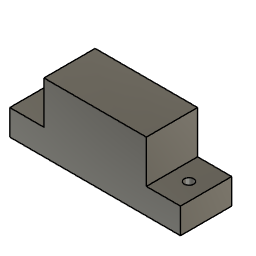
crank-holder (Autodesk Fusion 360 design; units mm, degrees)
Autodesk Fusion 360 part; units mm, degrees
sketch "main" plane through (0, 0, 0) normal (0, 1, 0) x (1, 0, 0) in component "crank-holder"
  line L0 (30, -20) -> (-30, -20)
  line L1 (-30, -20) -> (-30, 20)
  line L2 (-30, 20) -> (30, 20)
  line L3 (30, 20) -> (30, -20)
  line L4 (30, -20) -> (-30, 20) construction
  line L5 (-30, -20) -> (30, 20) construction
  circle A0 centre (0, 0) radius 4.425
  line L6 (-30, 20) -> (-50, 20) construction
  line L7 (-50, 20) -> (50, 20)
  line L8 (50, 20) -> (50, 5)
  line L9 (50, 5) -> (-50, 5)
  line L10 (-50, 5) -> (-50, 20)
  dimension "d1" = 60
  dimension "d2" = 40
  dimension "d3" = 8.85
  dimension "d4" = 20
  dimension "d5" = 100
  dimension "d6" = 15
  constraint horizontal L0
  constraint perpendicular L0 L1
  constraint parallel L0 L2
  constraint parallel L1 L3
  constraint coincident L4 A0.centre
  constraint coincident L5 A0.centre
  constraint coincident A0.centre origin
  constraint perpendicular L1 L6
  constraint horizontal L7
  constraint vertical L8
  constraint horizontal L9
  constraint vertical L10
  measures "d1" distance of L1.end L2.end
  measures "d2" distance of L0.end L1.end
  measures "d3" diameter of A0
  measures "d4" distance of L1.end L6.end
  measures "d5" distance of L6.end L7.end
  measures "d6" distance of L6.end L9.end
extrude "Extrude1" add sketch "main" against normal blind 30 contours L0 L1 L3 L9 | L1 L2 L3 L7 L9 | L3 L7 L8 L9 | L1 L7 L9 L10 | A0 in component "crank-holder"
extrude "Extrude2" add sketch "main" along normal blind 8.5 contours A0 in component "crank-holder"
sketch "screws" plane through (0, 0, -5) normal (0, 0, 1) x (-1, 0, 0) in component "crank-holder"
  line L0 (30, 0) -> (50, 0)
  line L1 (50, 0) -> (50, 30)
  line L2 (50, 30) -> (30, 30)
  line L3 (30, 30) -> (30, 0)
  line L4 (50, 0) -> (30, 30) construction
  line L5 (50, 30) -> (30, 0) construction
  line L6 (-50, 0) -> (-30, 30) construction
  line L7 (-50, 30) -> (-30, 0) construction
  circle A0 centre (40, 15) radius 2.75
  circle A1 centre (-40, 15) radius 2.75
  point P0 (-50, 0)
  point P1 (-30, 30)
  point P2 (-50, 30)
  point P3 (-30, 0)
  dimension "d11" = 5.5
  dimension "d12" = 5.5
  constraint coincident L0.end L1.start
  constraint coincident L2.end L3.start
  constraint coincident L1.end L2.start
  constraint coincident L0.start L3.end
  constraint coincident P0 L6.start
  constraint coincident P1 L6.end
  constraint coincident P2 L7.start
  constraint coincident P3 L7.end
  constraint midpoint L5 A0.centre
  constraint midpoint L7 A1.centre
  measures "d11" diameter of A0
  measures "d12" diameter of A1
extrude "Extrude3" cut sketch "screws" against normal blind 15 contours A0 | A1 in component "crank-holder"
component "crank-holder" placed x (1, 0, 0) y (0, 1, 0) z (0, 0, 1) at (0, 0, 0)
equation "d5 = 20 mm + 60 mm + 20 mm"
named bodies: "bearing-attachment"
